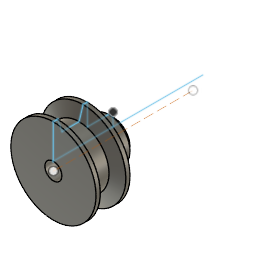
pully (Autodesk Fusion 360 design; units mm, degrees)
part number: 2026-04-15-09-51-42-530
Autodesk Fusion 360 part; units mm, degrees
sketch "Sketch1" plane through (0, 0, 0) normal (1, 0, 0) x (0, 1, 0)
  line L0 (-100, 30) -> (63.8964, 30) construction
  line L1 (-100, 40) -> (-30, 40)
  line L2 (-100, 40) -> (-100, 80)
  line L3 (-100, 80) -> (-95, 80)
  line L4 (-95, 80) -> (-89.6876, 65)
  line L5 (-89.6876, 65) -> (-69.7288, 65)
  line L6 (-69.7288, 65) -> (-65, 80)
  line L7 (-65, 80) -> (-60, 80)
  line L8 (-60, 80) -> (-60, 55)
  line L9 (-60, 55) -> (-35, 55)
  line L10 (-30, 50) -> (-30, 40)
  line L11 (-30, 40) -> (75.0845, 40)
  line L12 (-35, 55) -> (-30, 50)
  point P0 (-30, 55)
  dimension "d1" = 10
  dimension "d2" = 25
  dimension "d3" = 35
  dimension "d4" = 50
  dimension "d5" = 37
  dimension "d6" = 5
  dimension "d7" = 5
  dimension "d8" = 90
  dimension "d9" = 5
  dimension "d10" = 5
  dimension "d11" = 30
  dimension "d12" = 70
  constraint horizontal L0
  constraint horizontal L1
  constraint perpendicular L1 L2
  constraint perpendicular L2 L3
  constraint perpendicular L2 L5
  constraint parallel L5 L7
  constraint perpendicular L5 L8
  constraint perpendicular L8 L9
  constraint coincident L1 L11.end
  constraint collinear L3 L7
  constraint coincident P0 L9
  constraint coincident P0 L10
  measures "d1" distance of L0.end L1
  measures "d2" distance of L0.end L9
  measures "d3" distance of L0 L5
  measures "d4" distance of L0 L3
  measures "d5" angle of L4 L6
  measures "d6" distance of L2.end L3.end
  measures "d7" distance of L6.end L7.end
  measures "d8" angle of L1 L10
  measures "d9" distance of P0 L9.end
  measures "d10" distance of P0 L10.start
  measures "d11" distance of L3.end L6.end
  measures "d12" horizontal distance of L2.end P0
revolve "Revolve1" add sketch "Sketch1" angle 360 about axis through (0, -100, 30) along (0, 1, 0)
equation "d10 = d9"
